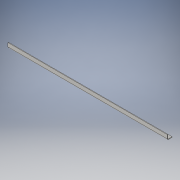
# Autodesk Inventor part: bar thing
Saved by Autodesk Inventor 2016 SP2 (Build 200236200, 236)
## iProperties
Created: 2018-01-17
Part Number: bar thing
Material: Generic
Document SubType Name: Sheet Metal
Designer: CAD
Density: 1 g/cm^3
Sheet Metal Rule: Default
Appearance: Default
Author: CAD
Autodesk Inventor part; units mm, degrees
ref_plane "YZ Plane" through (0, 0, 0) normal (1, 0, 0) x (0, 1, 0)
ref_plane "XZ Plane" through (0, 0, 0) normal (0, 1, 0) x (-1, 0, 0)
ref_plane "XY Plane" through (0, 0, 0) normal (0, 0, 1) x (1, 0, 0)
sketch "Sketch1" plane through (0, 0, 0) normal (0, 1, 0) x (-1, 0, 0)
  line L0 (0, 0) -> (0, -25.4)
  line L1 (0, 0) -> (819.15, 0)
  line L2 (0, -25.4) -> (819.15, -25.4)
  line L3 (819.15, -25.4) -> (819.15, 0)
  dimension "d1" = 819.15
  dimension "d2" = 25.4
  measures "d1" distance of L0.start L1.end
  measures "d2" distance of L0.start L0.end
sketch "Sketch3" plane through (-819.15, 0, 0) normal (0, 0, 1) x (1, 0, 0)
  line L0 (819.15, 3.175) -> (819.15, 25.4)
  line L1 (819.15, 25.4) -> (0, 25.4)
  line L2 (819.15, 0) -> (0, 0)
  line L3 (0, 25.4) -> (0, 3.175)
  line L4 (0, 3.175) -> (819.15, 3.175)
  line L5 (0, 3.175) -> (819.15, 3.175)
  line L6 (819.15, 0) -> (819.15, 3.175)
  line L7 (819.15, 3.175) -> (819.15, 0)
  dimension "d4" = 25.4
  measures "d4" distance of L2.start L0.end
extrude "Plate1" add sketch "Sketch1" along normal blind 3.175
sheet face with bend "Face2" sketch "Sketch3" thickness 3.175 toward (0, 0, -1) bend radius 3.175 relief straight relief width 3.175 relief depth 1.5875
bend "Bend1"
equation "\"d5\" = BendRadius"
equation "\"d6\" = BendReliefWidth"
equation "\"d8\" = MinimumRemnant"
equation "\"d7\" = BendReliefDepth"
equation "\"d9\" = BendRadius"
equation "\"BendRadius\" = Thickness"
equation "\"BendReliefWidth\" = Thickness"
equation "\"BendReliefDepth\" = 0.5 * Thickness"
equation "\"CornerReliefSize\" = 4 * Thickness"
equation "\"MinimumRemnant\" = 2 * Thickness"
equation "\"TransitionRadius\" = BendRadius"
equation "\"JacobiRadiusSize\" = BendRadius"
equation "\"GapSize\" = Thickness"
equation "\"d3\" = BendRadius"
equation "\"Thickness\" = 3.175"
body "Solid1"
